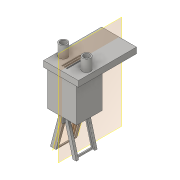
# Autodesk Inventor part: jtd_lid_auxiliary_electrode_2_2_20170428
Saved by Autodesk Inventor 2016 (Build 200138000, 138)
## iProperties
Created: 2017-04-21
Part Number: jtd_lid_auxiliary_electrode_2_2_20170428
Material: Generic
Document SubType Name: Modeling
Designer: Jonathan
Density: 1 g/cm^3
Appearance: Default
Author: Jonathan
Autodesk Inventor part; units mm, degrees
ref_plane "XZ Plane" through (0, 0, 0) normal (0, 1, 0) x (-1, 0, 0)
ref_plane "XY Plane" through (0, 0, 0) normal (0, 0, 1) x (1, 0, 0)
sketch "Sketch1" plane through (0, 0, 0) normal (0, 1, 0) x (-1, 0, 0)
  line L0 (15, -25) -> (-15, -25)
  line L1 (-15, -25) -> (-15, 25)
  line L2 (-15, 25) -> (15, 25)
  line L3 (15, 25) -> (15, -25)
  line L4 (15, -25) -> (-15, 25) construction
  line L5 (-15, -25) -> (15, 25) construction
  point P0 (0, 0)
  dimension "d0" = 30
  dimension "d1" = 50
  constraints: 12 end point, 2 midpoint, 2 parallel, 1 horizontal, 1 perpendicular
  measures "d0" distance of L1.end L2.end
  measures "d1" distance of L0.end L1.end
extrude "Main Lid" add sketch "Sketch1" against normal blind 5
sketch "Sketch2" plane through (0, -5, 0) normal (0, -1, 0) x (1, 0, 0)
  line L0 (15, 25) -> (-15, 25) projected
  line L1 (0, 25) -> (0, -25)
  line L2 (-15, -25) -> (15, -25) projected
  line L3 (12.5, 24) -> (-12.5, 24)
  line L4 (-12.5, 24) -> (-12.5, 2)
  line L5 (-12.5, 2) -> (12.5, 2)
  line L6 (12.5, 2) -> (12.5, 24)
  line L7 (12.5, 24) -> (-12.5, 2) construction
  line L8 (-12.5, 24) -> (12.5, 2) construction
  point P0 (0, 0)
  point P1 (0, 13)
  dimension "d4" = 25
  dimension "d5" = 22
  dimension "d7" = 1
  constraints: 14 end point, 4 midpoint, 2 parallel, 1 horizontal, 1 perpendicular, 1 point on line
  measures "d4" distance of L5.end L4.end
  measures "d5" distance of L5.end L3.start
  measures "d7" distance between parallel lines of L3 L0
extrude "Collection Chamber Exterior" add sketch "Sketch2" along normal blind 30
sketch "Sketch3" plane through (0, -35, 0) normal (0, -1, 0) x (1, 0, 0)
  line L0 (12.5, 2) -> (-12.5, 2) projected
  line L1 (0, 2) -> (0, 24)
  line L2 (-12.5, 24) -> (12.5, 24) projected
  line L3 (12.5, 24) -> (12.5, 2) projected
  line L4 (12.5, 13) -> (-12.5, 13)
  line L5 (-12.5, 2) -> (-12.5, 24) projected
  line L6 (11.5, 3) -> (2.5, 3)
  line L7 (2.5, 3) -> (2.5, 23)
  line L8 (2.5, 23) -> (11.5, 23)
  line L9 (11.5, 23) -> (11.5, 3)
  line L10 (-11.5, 3) -> (-2.5, 3)
  line L11 (-2.5, 3) -> (-2.5, 23)
  line L12 (-2.5, 23) -> (-11.5, 23)
  line L13 (-11.5, 23) -> (-11.5, 3)
  point P0 (0, 0)
  dimension "d10" = 9
  dimension "d11" = 20
  dimension "d12" = 1
  constraints: 20 end point, 4 midpoint, 4 symmetric about line, 2 parallel, 1 horizontal, 1 perpendicular, 1 other
  measures "d10" distance of L6.start L6.end
  measures "d11" distance of L8.end L6.start
  measures "d12" distance between parallel lines of L3 L9
extrude "Collection Volume" cut sketch "Sketch3" against normal up to surface (30 mm away) contours L11 L10 L13 L4 | L4 L13 L12 L11
mirror "Cathode Collection Vol" about plane through (0, 0, 0) normal (1, 0, 0) of "Collection Volume"
sketch "Sketch4" plane through (0, -35, 0) normal (0, -1, 0) x (1, 0, 0)
  line L0 (12.5, 24) -> (-12.5, 24) projected
  line L1 (0, 24) -> (0, 2)
  line L2 (-12.5, 2) -> (12.5, 2) projected
  line L3 (0.5, 24) -> (-0.5, 24)
  line L4 (-0.5, 24) -> (-0.5, 2)
  line L5 (-0.5, 2) -> (0.5, 2)
  line L6 (0.5, 2) -> (0.5, 24)
  point P0 (0, 0)
  dimension "d15" = 1
  constraints: 10 end point, 2 midpoint, 2 parallel, 2 point on line, 1 horizontal, 1 perpendicular, 1 other
  measures "d15" distance between parallel lines of L4 L6
extrude "Baffle" add sketch "Sketch4" along normal blind 5
sketch "Sketch5" plane through (0, -35, 0) normal (0, -1, 0) x (1, 0, 0)
  line L0 (12.5, 2) -> (12.5, 24) projected
  line L1 (12.5, 13) -> (-12.5, 13)
  line L2 (-12.5, 24) -> (-12.5, 2) projected
  line L3 (0.5, 2) -> (0.5, 24) projected
  line L4 (1.4121, 21) -> (0.5, 21)
  line L5 (0.5, 21) -> (0.5, 5)
  line L6 (0.5, 5) -> (1.4121, 5)
  line L7 (1.4121, 5) -> (1.4121, 21)
  line L8 (-12.5, 24) -> (12.5, 24) projected
  line L9 (0, 24) -> (0, 2)
  line L10 (12.5, 2) -> (-12.5, 2) projected
  line L11 (-1.4121, 21) -> (-0.5, 21)
  line L12 (-0.5, 21) -> (-0.5, 5)
  line L13 (-0.5, 5) -> (-1.4121, 5)
  line L14 (-1.4121, 5) -> (-1.4121, 21)
  point P0 (0, 0)
  dimension "d18" = 16
  constraints: 20 end point, 4 midpoint, 4 symmetric about line, 2 parallel, 1 horizontal, 1 perpendicular, 1 point on line, 1 other
  measures "d18" distance of L6.end L4.start
extrude "Electrode Slits" cut sketch "Sketch5" against normal through all contours L7 L6 L3 L1 | L1 L3 L4 L7 | L12 L13 L14 L1 | L1 L14 L11 L12
sketch "Sketch6" plane through (0, 0, 0) normal (0, 1, 0) x (1, 0, 0)
  line L0 (15, -25) -> (-15, -25) projected
  line L1 (0, -25) -> (0, 25)
  line L2 (-15, 25) -> (15, 25) projected
  line L3 (-2.5, -23) -> (-2.5, -3) projected
  line L4 (-2.5, -13) -> (-11.5, -13)
  line L5 (-11.5, -3) -> (-11.5, -23) projected
  line L6 (-11.5, -23) -> (-2.5, -23) projected
  line L7 (-2.5, -3) -> (-11.5, -3) projected
  circle A0 centre (-10, -13) radius 1.5
  circle A1 centre (10, -13) radius 1.5
  point P0 (0, 0)
  dimension "d24" = 3
  constraints: 4 end point, 4 midpoint, 1 centre point, 1 horizontal alignment, 1 point on line, 1 symmetric about line, 3 other
extrude "Gas Collection Holes" cut sketch "Sketch6" against normal through all contours A0 L4 | L4 A0 | A1
sketch "Sketch7" plane through (0, 0, 0) normal (0, 1, 0) x (1, 0, 0)
  circle A0 centre (-10, -13) radius 2.5
  circle A1 centre (-10, -13) radius 1.5 projected
  circle A2 centre (-10, -13) radius 3.5
  line L0 (15, -25) -> (-15, -25) projected
  line L1 (0, -25) -> (0, -2)
  line L2 (-0.5, -2) -> (0.5, -2) projected
  circle A3 centre (10, -13) radius 2.5
  circle A4 centre (10, -13) radius 3.5
  point P0 (0, 0)
  dimension "d27" = 5
  dimension "d28" = 1
  constraints: 4 centre point, 2 end point, 2 midpoint, 2 symmetric about line, 1 coincident, 1 concentric, 2 other
  measures "d27" diameter of A0
  measures "d28" radial gap between concentric circles of A0 A2
extrude "Gas Collection Ports" add sketch "Sketch7" along normal blind 10 contours A2 | A4
sketch "Sketch8" plane through (0, -35, 0) normal (0, -1, 0) x (1, 0, 0)
  line L0 (-2.4121, 21) -> (-3.3242, 21)
  line L1 (-3.3242, 21) -> (-3.3242, 5)
  line L2 (-3.3242, 5) -> (-2.4121, 5)
  line L3 (-2.4121, 5) -> (-2.4121, 21)
  line L4 (-0.5, 5) -> (-1.4121, 5) projected
  line L5 (-1.4121, 21) -> (-0.5, 21) projected
  line L6 (-1.4121, 5) -> (-1.4121, 21) projected
  point P0 (0, 0)
  dimension "d31" = 1
  constraints: 8 end point, 3 collinear, 2 parallel, 1 horizontal, 1 perpendicular
  measures "d31" distance between parallel lines of L3 L6
extrude "Aux elect hole" cut sketch "Sketch8" against normal blind 40
sketch "Sketch9" plane through (0, -35, 0) normal (0, -1, 0) x (1, 0, 0)
  line L0 (-2.4121, 21) -> (-3.3242, 21) projected
  line L1 (-2.5, 5) -> (-3.3242, 5) projected
  line L2 (-2.4121, 21) -> (-3.3242, 21)
  line L3 (-3.3242, 21) -> (-3.3242, 5)
  line L4 (-3.3242, 5) -> (-2.4121, 5)
  line L5 (-2.4121, 5) -> (-2.4121, 21)
  line L6 (-2.4121, 22) -> (-4.3242, 22)
  line L7 (-4.3242, 22) -> (-4.3242, 4)
  line L8 (-4.3242, 4) -> (-2.4121, 4)
  line L9 (-2.4121, 4) -> (-2.4121, 22)
  point P0 (0, 0)
  dimension "d34" = 1
  dimension "d35" = 1
  dimension "d36" = 1
  constraints: 16 end point, 4 parallel, 2 horizontal, 2 perpendicular, 1 collinear
  measures "d34" distance between parallel lines of L8 L4
  measures "d35" distance between parallel lines of L0 L6
  measures "d36" distance between parallel lines of L7 L3
extrude "Aux elect cover" add sketch "Sketch9" against normal up to surface (35 mm away) contours L0 L3 L1 L4 L9 L8 L7 L6
sketch "Sketch11" plane through (0, -35, 0) normal (0, -1, 0) x (1, 0, 0)
  line L0 (2.5, 3) -> (2.5, 23) projected
  line L1 (2.5, 13) -> (-4.3242, 13)
  line L2 (-4.3242, 22) -> (-4.3242, 4) projected
  line L3 (0.5, 24) -> (0.5, 21) projected
  line L4 (0.5, 21) -> (0.5, 19.9628)
  line L5 (0.5, 2) -> (0.5, 24) projected
  line L6 (-0.5, 19.9628) -> (-0.5, 22)
  line L7 (-0.5, 22) -> (2.4121, 22)
  line L8 (2.4121, 22) -> (2.4121, 19.9628)
  line L9 (2.4121, 19.9628) -> (1.4121, 19.9628)
  line L10 (1.4121, 21) -> (1.4121, 5) projected
  line L11 (1.4121, 21) -> (0.5, 21)
  line L12 (0.5, 19.9628) -> (-0.5, 19.9628)
  line L13 (1.4121, 21) -> (1.4121, 19.9628)
  line L14 (0.5, 5) -> (0.5, 6.0372)
  line L15 (-0.5, 6.0372) -> (-0.5, 4)
  line L16 (-0.5, 4) -> (2.4121, 4)
  line L17 (2.4121, 4) -> (2.4121, 6.0372)
  line L18 (2.4121, 6.0372) -> (1.4121, 6.0372)
  line L19 (1.4121, 5) -> (0.5, 5)
  line L20 (0.5, 6.0372) -> (-0.5, 6.0372)
  line L21 (1.4121, 5) -> (1.4121, 6.0372)
  point P0 (0, 0)
  dimension "d39" = 1
  dimension "d40" = 1
  constraints: 34 end point, 7 symmetric about line, 4 perpendicular, 2 collinear, 2 midpoint, 2 point on line, 1 parallel, 1 vertical
  measures "d39" distance of L8.end L9.end
  measures "d40" distance between parallel lines of L7 L11
sketch "Sketch12" plane through (-12.5, -5, 24) normal (0, 0, 1) x (1, 0, 0)
  line L0 (13, -30) -> (20.7646, -58.9778)
  line L1 (12.5, 5) -> (12.5, -30)
  dimension "d41" = 30
  dimension "d42" = 15
  constraints: 4 end point, 1 vertical
  measures "d41" distance of L0.start L0.end
  measures "d42" angle of L1 L0
sweep "Cathode Rail" add profiles "Sketch11" path "Sketch12" path curves L0 contours L10 L11 L3 L7 L8 L9 | L18 L17 L16 L5 L19 L10 | L5 L16 L15 L20 | L12 L6 L7 L3 L4
sketch "Sketch14" plane through (0, -35, 0) normal (0, -1, 0) x (1, 0, 0)
  line L0 (-2.4121, 21) -> (-2.4121, 5) projected
  line L1 (-2.4121, 21) -> (-2.4121, 20)
  line L2 (-4.3242, 20) -> (-4.3242, 22)
  line L3 (0.5, 24) -> (0.5, 22) projected
  line L4 (-4.3242, 22) -> (0.5, 22)
  line L5 (0.5, 22) -> (0.5, 20)
  line L6 (0.5, 2) -> (0.5, 24) projected
  line L7 (-0.5, 20) -> (-0.5, 21)
  line L8 (-1.4121, 5) -> (-1.4121, 21) projected
  line L9 (-0.5, 21) -> (-1.4121, 21)
  line L10 (-2.4121, 20) -> (-1.4121, 20)
  line L11 (-1.4121, 21) -> (-1.4121, 20)
  line L12 (-2.4121, 21) -> (-3.3242, 21)
  line L13 (-3.3242, 21) -> (-3.3242, 20)
  line L14 (-3.3242, 5) -> (-3.3242, 21) projected
  line L15 (-3.3242, 20) -> (-4.3242, 20)
  line L16 (0.5, 20) -> (-0.5, 20)
  line L17 (0.5, 22) -> (0.5, 20)
  line L18 (-0.5, 21) -> (-0.5, 20)
  line L19 (-0.5, 24) -> (-0.5, 2) projected
  line L20 (-4.3242, 22) -> (-4.3242, 4) projected
  line L21 (-4.3242, 13) -> (0.5, 13)
  line L22 (-2.4121, 5) -> (-2.4121, 6)
  line L23 (-4.3242, 6) -> (-4.3242, 4)
  line L24 (-4.3242, 4) -> (0.5, 4)
  line L25 (0.5, 4) -> (0.5, 6)
  line L26 (-0.5, 6) -> (-0.5, 5)
  line L27 (-0.5, 5) -> (-1.4121, 5)
  line L28 (-2.4121, 6) -> (-1.4121, 6)
  line L29 (-1.4121, 5) -> (-1.4121, 6)
  line L30 (-2.4121, 5) -> (-3.3242, 5)
  line L31 (-3.3242, 5) -> (-3.3242, 6)
  line L32 (-3.3242, 6) -> (-4.3242, 6)
  line L33 (0.5, 6) -> (-0.5, 6)
  line L34 (0.5, 4) -> (0.5, 6)
  line L35 (-0.5, 5) -> (-0.5, 6)
  point P0 (0, 0)
  dimension "d45" = 1
  dimension "d47" = 1
  dimension "d48" = 1
  constraints: 58 end point, 8 symmetric about line, 4 horizontal, 4 point on line, 3 collinear, 2 midpoint, 1 parallel
  measures "d45" distance of L8.end L10.end
  measures "d47" distance of L7.end L7.start
  measures "d48" distance of L12.end L13.end
sketch "Sketch16" plane through (-12.5, -5, 24) normal (0, 0, 1) x (1, 0, 0)
  line L0 (12, -30) -> (12, -35) projected
  line L1 (12, -30) -> (4.2354, -58.9778)
  line L2 (12.5, 5) -> (12.5, -30)
  dimension "d53" = 30
  dimension "d54" = 15
  constraints: 4 end point, 1 vertical
  measures "d53" distance of L0.start L1.end
  measures "d54" angle of L2 L1
surface extrude "ExtrusionSrf1" sketch "Sketch16" against normal up to surface (22 mm away) shown yes curves L0 L1
sketch "Sketch17" plane through (-0.5, -35, 24) normal (0.9659258, -0.258819, 0) x (0, 0, -1)
  line L0 (19.6592, 0) -> (19.6592, -30)
  line L1 (22, 0) -> (19, 0) projected
  point P0 (24, 33.9368)
  dimension "d57" = 30
  constraints: 2 end point, 1 point on line, 1 vertical
  measures "d57" distance of L0.start L0.end
sweep "Sweep2" add profiles "Sketch14" path "Sketch17" path curves L0 contours L12 L13 L15 L2 L4 L19 L9 L8 L10 L0 | L28 L8 L27 L19 L24 L20 L32 L14 L30 L0 | L19 L4 L5 L16 L7 | L33 L6 L24 L19
sketch "Sketch18" plane through (-8.2646, -63.9778, 6) normal (0, 0, 1) x (1, 0, 0)
  line L0 (7.7646, 28.9778) -> (0, 0) projected
  line L1 (7.7646, 25.2457) -> (1, 0) projected
  line L2 (0, 0) -> (1, 0)
  line L3 (1, 0) -> (1.2588, 0.9659)
  line L4 (1.2588, 0.9659) -> (0.2588, 0.9659)
  line L5 (0.2588, 0.9659) -> (0, 0)
  point P0 (8.2646, 63.9778)
  dimension "d60" = 1
  constraints: 8 end point, 2 parallel, 2 point on line, 1 horizontal
  measures "d60" distance of L1.end L3.end
extrude "Lower anode support" add sketch "Sketch18" along normal up to surface (14 mm away)
sketch "Sketch19" plane through (7.2646, -63.9778, 6.0372) normal (0, 0, 1) x (1, 0, 0)
  line L0 (-6.7646, 25.2457) -> (0, 0) projected
  line L1 (1, 0) -> (0, 0)
  line L2 (0, 0) -> (-0.2588, 0.9659)
  line L3 (-0.2588, 0.9659) -> (0.7412, 0.9659)
  line L4 (-6.7646, 28.9778) -> (1, 0) projected
  line L5 (1, 0) -> (0.7412, 0.9659)
  line L6 (1, 0) -> (0, 0) projected
  point P0 (-7.2646, 63.9778)
  dimension "d63" = 1
  constraints: 8 end point, 2 point on line, 1 collinear, 1 horizontal, 1 parallel
  measures "d63" distance of L0.end L2.end
extrude "Lower Cathode Support" add sketch "Sketch19" along normal up to surface (13.9256 mm away)
body "Solid1"
body "Srf1"
